# Autodesk Inventor part: RPi_BeamProfiler.kicad_pcb_Outline
Saved by Autodesk Inventor 2016 (Build 200138000, 138)
## iProperties
Created: 2017-03-06
Part Number: RPi_BeamProfiler.kicad_pcb_Outline
Material: Generic
Document SubType Name: Modeling
Designer: James
Density: 1 g/cm^3
Appearance: Board Outline
Author: James
Autodesk Inventor part; units mm, degrees
ref_plane "YZ Plane" through (0, 0, 0) normal (1, 0, 0) x (0, 1, 0)
ref_plane "XZ Plane" through (0, 0, 0) normal (0, 1, 0) x (-1, 0, 0)
ref_plane "XY Plane" through (0, 0, 0) normal (0, 0, 1) x (1, 0, 0)
sketch "Sketch1" plane through (0, 0, 0) normal (0, 0, 1) x (1, 0, 0)
  line L0 (26.67, 27.559) -> (-26.67, 27.559)
  line L1 (-26.67, 27.559) -> (-26.67, -27.559)
  line L2 (-26.67, -27.559) -> (26.67, -27.559)
  line L3 (26.67, -27.559) -> (26.67, 27.559)
  line L4 (-12.042, -18.685) -> (-12.042, -20.685)
  arc A0 (-13.042, -20.685) -> (-12.042, -20.685) centre (-12.542, -20.685) ccw
  line L5 (-13.042, -20.685) -> (-13.042, -18.685)
  arc A1 (-12.042, -18.685) -> (-13.042, -18.685) centre (-12.542, -18.685) ccw
  line L6 (-18.042, -18.685) -> (-18.042, -20.685)
  arc A2 (-19.042, -20.685) -> (-18.042, -20.685) centre (-18.542, -20.685) ccw
  line L7 (-19.042, -20.685) -> (-19.042, -18.685)
  arc A3 (-18.042, -18.685) -> (-19.042, -18.685) centre (-18.542, -18.685) ccw
  line L8 (-14.542, -24.885) -> (-16.542, -24.885)
  arc A4 (-16.542, -23.885) -> (-16.542, -24.885) centre (-16.542, -24.385) ccw
  line L9 (-16.542, -23.885) -> (-14.542, -23.885)
  arc A5 (-14.542, -24.885) -> (-14.542, -23.885) centre (-14.542, -24.385) ccw
  circle A6 centre (8.636, -5.461) radius 0.4
  circle A7 centre (6.136, -5.461) radius 0.4
  circle A8 centre (-18.288, 5.033) radius 0.5
  circle A9 centre (-18.288, 10.033) radius 0.5
  circle A10 centre (11.938, 23.455) radius 0.4
  circle A11 centre (11.938, 20.955) radius 0.4
  circle A12 centre (-12.192, -6.985) radius 0.7
  circle A13 centre (-12.192, -1.905) radius 0.7
  circle A14 centre (-3.302, -1.905) radius 0.4065
  circle A15 centre (-3.302, -6.985) radius 0.4065
  circle A16 centre (-13.208, 24.511) radius 0.5
  circle A17 centre (-15.748, 24.511) radius 0.5
  circle A18 centre (-18.288, 24.511) radius 0.5
  circle A19 centre (-20.828, 24.511) radius 0.5
  circle A20 centre (-24.13, 19.431) radius 0.5
  circle A21 centre (-24.13, 16.891) radius 0.5
  circle A22 centre (-21.59, -8.509) radius 0.4
  circle A23 centre (-21.59, -0.889) radius 0.4
  circle A24 centre (6.858, -15.875) radius 0.5
  circle A25 centre (5.158, -19.575) radius 0.5
  circle A26 centre (3.458, -15.875) radius 0.5
  circle A27 centre (1.758, -19.575) radius 0.5
  circle A28 centre (0.058, -15.875) radius 0.5
  circle A29 centre (20.574, 24.765) radius 0.5
  circle A30 centre (23.114, 24.765) radius 0.5
  circle A31 centre (20.574, 22.225) radius 0.5
  circle A32 centre (23.114, 22.225) radius 0.5
  circle A33 centre (20.574, 19.685) radius 0.5
  circle A34 centre (23.114, 19.685) radius 0.5
  circle A35 centre (20.574, 17.145) radius 0.5
  circle A36 centre (23.114, 17.145) radius 0.5
  circle A37 centre (20.574, 14.605) radius 0.5
  circle A38 centre (23.114, 14.605) radius 0.5
  circle A39 centre (20.574, 12.065) radius 0.5
  circle A40 centre (23.114, 12.065) radius 0.5
  circle A41 centre (20.574, 9.525) radius 0.5
  circle A42 centre (23.114, 9.525) radius 0.5
  circle A43 centre (20.574, 6.985) radius 0.5
  circle A44 centre (23.114, 6.985) radius 0.5
  circle A45 centre (20.574, 4.445) radius 0.5
  circle A46 centre (23.114, 4.445) radius 0.5
  circle A47 centre (20.574, 1.905) radius 0.5
  circle A48 centre (23.114, 1.905) radius 0.5
  circle A49 centre (20.574, -0.635) radius 0.5
  circle A50 centre (23.114, -0.635) radius 0.5
  circle A51 centre (20.574, -3.175) radius 0.5
  circle A52 centre (23.114, -3.175) radius 0.5
  circle A53 centre (20.574, -5.715) radius 0.5
  circle A54 centre (23.114, -5.715) radius 0.5
  circle A55 centre (20.574, -8.255) radius 0.5
  circle A56 centre (23.114, -8.255) radius 0.5
  circle A57 centre (20.574, -10.795) radius 0.5
  circle A58 centre (23.114, -10.795) radius 0.5
  circle A59 centre (20.574, -13.335) radius 0.5
  circle A60 centre (23.114, -13.335) radius 0.5
  circle A61 centre (20.574, -15.875) radius 0.5
  circle A62 centre (23.114, -15.875) radius 0.5
  circle A63 centre (20.574, -18.415) radius 0.5
  circle A64 centre (23.114, -18.415) radius 0.5
  circle A65 centre (20.574, -20.955) radius 0.5
  circle A66 centre (23.114, -20.955) radius 0.5
  circle A67 centre (20.574, -23.495) radius 0.5
  circle A68 centre (23.114, -23.495) radius 0.5
  circle A69 centre (5.08, 20.447) radius 0.4
  circle A70 centre (-7.62, 20.447) radius 0.4
  circle A71 centre (5.08, 17.907) radius 0.4
  circle A72 centre (-7.62, 17.907) radius 0.4
  circle A73 centre (5.08, 15.367) radius 0.4
  circle A74 centre (-7.62, 15.367) radius 0.4
  circle A75 centre (5.08, 12.827) radius 0.4
  circle A76 centre (-7.62, 12.827) radius 0.4
  circle A77 centre (5.08, 10.287) radius 0.4
  circle A78 centre (-7.62, 10.287) radius 0.4
  circle A79 centre (5.08, 7.747) radius 0.4
  circle A80 centre (-7.62, 7.747) radius 0.4
  circle A81 centre (5.08, 5.207) radius 0.4
  circle A82 centre (-7.62, 5.207) radius 0.4
  circle A83 centre (5.08, 2.667) radius 0.4
  circle A84 centre (-7.62, 2.667) radius 0.4
  constraints: 85 centre point, 20 end point, 12 point on circle
extrude "RPi_BeamProfiler.kicad_pcb_Outline" add sketch "Sketch1" along normal blind 1.6
body "Solid1"
